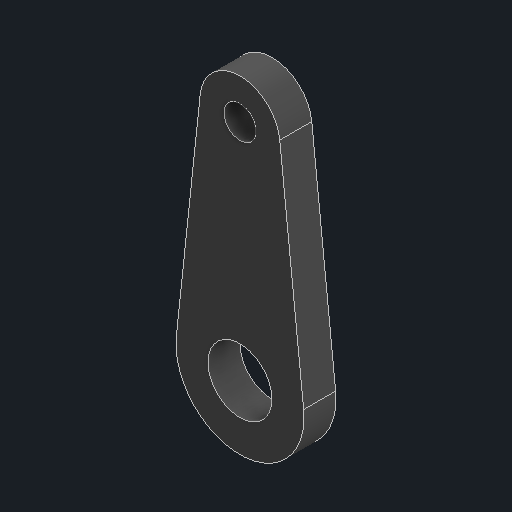
# Autodesk Inventor part: servo_arm
Saved by Autodesk Inventor 2022.2 (Build 262287010, 287A)
## iProperties
Created: 2022-03-30
Part Number: servo_arm
Material: Generic
Document SubType Name: Modeling
Designer: kardo
Density: 1 g/cm^3
Appearance: Dark Plastic
Author: kardo
Autodesk Inventor part; units mm, degrees
ref_plane "YZ Plane" through (0, 0, 0) normal (1, 0, 0) x (0, 1, 0)
ref_plane "XZ Plane" through (0, 0, 0) normal (0, 1, 0) x (-1, 0, 0)
ref_plane "XY Plane" through (0, 0, 0) normal (0, 0, 1) x (1, 0, 0)
derived "parameters_powertrain.ipt"
sketch "sk_base" plane through (0, 0, 0) normal (0, 0, 1) x (1, 0, 0)
  arc A0 (-3.977, 0.4286) -> (3.977, 0.4286) centre (0, 0) ccw
  line L0 (-3.977, 0.4286) -> (-2.4856, 14.2679)
  line L1 (2.4856, 14.2679) -> (3.977, 0.4286)
  arc A1 (2.4856, 14.2679) -> (-2.4856, 14.2679) centre (0, 14) ccw
  line L2 (-5.6, 0) -> (5.6, 0) construction
  line L3 (0, -8.1) -> (0, 20.6) construction
  dimension "d0" = 14
  dimension "d13" = 8
  dimension "d14" = 5
  constraints: 4 end point, 4 point on circle, 4 tangent, 2 centre point, 2 coincident, 2 point on line, 1 midpoint
  measures "d0" distance of point (0, 0) A1.centre
  measures "d13" diameter of A0
  measures "d14" diameter of A1
extrude "thicken" add sketch "sk_base" against normal blind 2
hole "shaft_hole" at (0, 0, 0) direction (0, 0, -1) diameter 4 end through all
hole "joint_hole" at (0, 14, 0) direction (0, 0, -1) diameter 2 end through all
equation "\"d0\" = servo_arm_length"
equation "\"servo_arm_length\" = 14"
body "Solid1"
